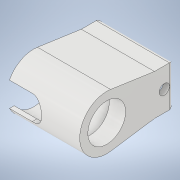
# Autodesk Inventor part: tail_encoder
Saved by Autodesk Inventor 2020 (Build 240168000, 168)
## iProperties
Created: 2018-05-10
Part Number: tail_encoder
Material: Generic
Document SubType Name: Modeling
Designer: stedrock
Density: 1 g/cm^3
Appearance: Default
Mass: 13.8851 g
Surface Area: 94.7181 cm^2
Volume: 13.8851 cm^3
PCB_thickness: 1.650 mm
wall: 3.000 mm
PCB_height: 3.460 mm
Author: stedrock
Autodesk Inventor part; units mm, degrees
sketch "Sketch1" plane through (0, 0, 0) normal (0, 0, 1) x (1, 0, 0)
  line L0 (-9.42, -6.99) -> (9.42, -6.99)
  line L1 (9.42, -6.99) -> (9.42, 6.99)
  line L2 (9.42, 6.99) -> (-9.42, 6.99)
  line L3 (-9.42, 6.99) -> (-9.42, -6.99)
  line L4 (-9.42, -6.99) -> (9.42, 6.99) construction
  line L5 (9.42, -6.99) -> (-9.42, 6.99) construction
  line L6 (0, 0) -> (-12.7572, 0) construction
  line L7 (-4.42, -2.5) -> (1.88, -2.5)
  line L8 (1.88, -2.5) -> (1.88, 2.5)
  line L9 (1.88, 2.5) -> (-4.42, 2.5)
  line L10 (-4.42, 2.5) -> (-4.42, -2.5)
  line L11 (-4.42, -2.5) -> (1.88, 2.5) construction
  line L12 (1.88, -2.5) -> (-4.42, 2.5) construction
  line L13 (-12.42, -9.99) -> (23.42, -9.99)
  line L14 (23.42, -9.99) -> (23.42, 9.99)
  line L15 (23.42, 9.99) -> (-12.42, 9.99)
  line L16 (-12.42, 9.99) -> (-12.42, -9.99)
  line L17 (-12.42, -9.99) -> (23.42, 9.99) construction
  line L18 (23.42, -9.99) -> (-12.42, 9.99) construction
  line L19 (-9.42, 6.99) -> (-7.42, 6.99)
  line L20 (-7.42, 6.99) -> (-7.42, -6.99)
  line L21 (-7.42, -6.99) -> (-9.42, -6.99)
  line L22 (-9.42, -6.99) -> (-9.42, 6.99)
  line L23 (-9.42, 6.99) -> (5.42, 6.99)
  line L24 (5.42, 6.99) -> (5.42, 4.99)
  line L25 (5.42, 4.99) -> (-9.42, 4.99)
  line L26 (-9.42, 4.99) -> (-9.42, 6.99)
  line L27 (-9.42, -6.99) -> (5.42, -6.99)
  line L28 (5.42, -6.99) -> (5.42, -4.99)
  line L29 (5.42, -4.99) -> (-9.42, -4.99)
  line L30 (-9.42, -4.99) -> (-9.42, -6.99)
  line L31 (-1.27, 0) -> (31.11, 0) construction
  line L32 (9.42, 6.99) -> (20.42, 6.99)
  line L33 (20.42, 6.99) -> (20.42, -6.99)
  line L34 (20.42, -6.99) -> (9.42, -6.99)
  line L35 (9.42, -6.99) -> (9.42, 6.99)
  line L36 (9.42, 6.99) -> (20.42, -6.99) construction
  line L37 (20.42, 6.99) -> (9.42, -6.99) construction
  circle A0 centre (-1.27, 0) radius 1.5
  line L38 (19.42, -6.99) -> (19.42, 6.99)
  point P0 (5.5, 0)
  point P1 (14.92, 0)
  dimension "d0" = 18.84
  dimension "d1" = 13.98
  dimension "d2" = 6.3
  dimension "d3" = 5
  dimension "d4" = 11.3
  dimension "d5" = 13.84
  dimension "d10" = 3
  dimension "d11" = 3
  dimension "d12" = 14
  dimension "d17" = 2
  dimension "d18" = 2
  dimension "d19" = 4
  dimension "d20" = 2
  dimension "d21" = 4
  dimension "d22" = 3
  dimension "d25" = 3
  dimension "d47" = 10
  constraints: 78 end point, 14 parallel, 9 midpoint, 8 perpendicular, 7 horizontal, 6 point on line, 1 centre point, 1 coincident, 1 vertical
  measures "d0" distance of L2.end L1.end
  measures "d1" distance of L1.end L0.end
  measures "d2" distance of L9.end L8.end
  measures "d3" distance of L7.end L8.end
  measures "d4" distance between parallel lines of L8 L3
  measures "d5" distance between parallel lines of L1 L10
  measures "d10" distance between parallel lines of L2 L15
  measures "d11" distance between parallel lines of L3 L16
  measures "d12" distance between parallel lines of L14 L1
  measures "d17" distance between parallel lines of L20 L3
  measures "d18" distance of L23.end L24.end
  measures "d19" distance between parallel lines of L1 L24
  measures "d20" distance between parallel lines of L27 L29
  measures "d21" distance between parallel lines of L1 L28
  measures "d22" distance between parallel lines of L14 L33
  measures "d25" diameter of A0
  measures "d47" distance between parallel lines of L38 L35
extrude "top" add sketch "Sketch1" against normal blind 7 contours L16 L15 L14 L13
extrude "bottom" add sketch "Sketch1" along normal blind 2.31 contours L3 L29 L20 L0 | L20 L29 L28 L0 | L3 L25 L20 L29 | L3 L2 L20 L25 | L20 L2 L24 L25 | L38 L32 L33 L34 | L16 L15 L14 L13
ref_plane "Work Plane1" through (23.42, 9.99, 0) normal (1, 0, 0) x (0, 1, 0)
sketch "Sketch2" plane through (23.42, 9.99, 0) normal (1, 0, 0) x (0, 1, 0)
  line L0 (-9.99, 0) -> (-9.99, 39.738) construction
  circle A0 centre (-9.99, 25.712) radius 9.25
  circle A1 centre (-9.99, 25.712) radius 13.25
  line L1 (-19.98, 0) -> (0, 0) projected
  line L2 (-19.98, 2.31) -> (0, 2.31) projected
  line L3 (0, 2.31) -> (3.1224, 23.8075)
  line L4 (-19.98, 2.31) -> (-23.1024, 23.8075)
  line L5 (-6.699, 7.9835) -> (-13.281, 7.9835) construction
  line L6 (-6.699, 10.4835) -> (-13.281, 10.4835)
  line L7 (-13.281, 5.4835) -> (-6.699, 5.4835)
  arc A2 (-6.699, 5.4835) -> (-6.699, 10.4835) centre (-6.699, 7.9835) ccw
  arc A3 (-13.281, 10.4835) -> (-13.281, 5.4835) centre (-13.281, 7.9835) ccw
  circle A4 centre (-9.99, -2.5) radius 2.5
  point P0 (-9.99, 7.9835)
  dimension "d26" = 18.5
  dimension "d27" = 26.5
  dimension "d30" = 23.402
  dimension "d33" = 5
  dimension "d43" = 5
  dimension "d44" = 2.5
  constraints: 14 end point, 6 point on circle, 6 tangent, 5 centre point, 3 point on line, 1 coincident, 1 midpoint, 1 parallel, 1 perpendicular, 1 vertical
  measures "d26" diameter of A0
  measures "d27" diameter of A1
  measures "d30" distance from line of A0.centre L2
  measures "d33" diameter of A3
  measures "d43" diameter of A4
  measures "d44" distance from line of L1 A4.centre
extrude "holder" add sketch "Sketch2" against normal blind 8 contours A1 | A1 L3 L2 L4 | A2 L7 A3 L6
sketch "Sketch4" plane through (15.42, 9.99, 0) normal (-1, 0, 0) x (0, 0, 1)
  circle A0 centre (25.712, -9.99) radius 9.25 projected
  line L0 (23.8075, 3.1224) -> (2.31, 0) projected
  line L1 (2.31, -19.98) -> (23.8075, -23.1024) projected
  circle A1 centre (25.712, -9.99) radius 11.25
  line L2 (2.31, -19.98) -> (2.31, 0) projected
  arc A2 (23.8075, -23.1024) -> (23.8075, 3.1224) centre (25.712, -9.99) ccw projected
  line L3 (2.31, 0) -> (2.31, -19.98) projected
  line L4 (2.31, -16.9485) -> (19.65, -19.4671)
  line L5 (2.31, -3.0315) -> (19.65, -0.5129)
  circle A3 centre (25.712, -9.99) radius 13.25 projected
  line L6 (12.462, -1.5569) -> (12.462, -18.4231)
  point P0 (0, -9.99)
  point P1 (2.31, -2.0103)
  point P2 (24.5722, 1.2021)
  point P3 (2.31, -18.1795)
  point P4 (29.9517, -20.4105)
  dimension "d34" = 22.5
  dimension "d41" = 3
  dimension "d42" = 3
  constraints: 6 end point, 6 point on line, 4 point on circle, 2 parallel, 1 centre point, 1 coincident, 1 tangent, 1 vertical
  measures "d34" diameter of A1
  measures "d41" distance between parallel lines of L4 L1
  measures "d42" distance between parallel lines of L0 L5
extrude "holder2" add sketch "Sketch4" along normal up to surface (27.84 mm away) contours A3 L5 L2 L0 | A2 A3 L4 A1 L5 | A3 L6 L5 | L5 A1 L4 A3 | L1 L2 L4 A3 | A3 L4 L6
ref_plane "Work Plane2" through (0, 0, 42.8625) normal (0, 0, 1) x (1, 0, 0)
sketch "Sketch5" plane through (0, 0, 42.8625) normal (0, 0, 1) x (1, 0, 0)
  line L0 (-25.4872, 0) -> (-1.2329, 0) construction
  line L1 (-25.4872, -6) -> (-1.2329, -6)
  line L2 (-1.2329, 6) -> (-25.4872, 6)
  arc A0 (-25.4872, 6) -> (-25.4872, -6) centre (-25.4872, 0) ccw
  arc A1 (-1.2329, -6) -> (-1.2329, 6) centre (-1.2329, 0) ccw
  point P0 (0, 0)
  point P1 (-13.3601, 0)
  dimension "d38" = 12
  constraints: 8 end point, 4 point on circle, 4 tangent, 2 centre point, 1 horizontal, 1 midpoint, 1 parallel, 1 point on line
  measures "d38" diameter of A1
extrude "bottom hole" cut sketch "Sketch5" against normal blind 33.35
extrude "cable hole" cut sketch "Sketch2" against normal up to next contours A4
fillet "Fillet1" radius 2 4 edges at (5.5, 9.99, -7) (23.42, 0, -7) (5.5, -9.99, -7) (-12.42, 0, -7)
ref_plane "trim plane" through (-12.42, 9.99, 2.31) normal (0, 0, 1) x (1, 0, 0)
ref_plane "Work Plane4" through (47.625, 0, 0) normal (1, 0, 0) x (0, 1, 0)
sketch "split sketch" plane through (47.625, 0, 0) normal (1, 0, 0) x (0, 1, 0)
  line L0 (9.99, -5) -> (0, -5) projected
  line L1 (9.99, -5) -> (9.99, 2.31) projected
  line L2 (9.99, 2.31) -> (13.1124, 23.8075) projected
  arc A0 (13.1124, 23.8075) -> (-13.1124, 23.8075) centre (0, 25.712) ccw projected
  line L3 (-13.1124, 23.8075) -> (-9.99, 2.31) projected
  line L4 (-9.99, -5) -> (-9.99, 2.31) projected
  circle A1 centre (0, -2.5) radius 2.5 projected
  circle A2 centre (0, 25.712) radius 9.25 projected
  line L5 (9.99, -5) -> (9.99, 2.31) projected
  line L6 (-9.99, 2.31) -> (-7.7245, 2.31) projected
  line L7 (9.99, 2.31) -> (-9.99, 2.31)
  line L8 (9.99, 2.31) -> (-9.99, 2.31) projected
  line L9 (7.99, 2.31) -> (-7.99, 2.31)
  line L10 (-7.99, 2.31) -> (-7.99, -12.786)
  line L11 (-7.99, -12.786) -> (7.99, -12.786)
  line L12 (7.99, -12.786) -> (7.99, 2.31)
  line L13 (26.885, -21.7939) -> (-23.4802, -21.7939)
  line L14 (-23.4802, -21.7939) -> (-23.4802, 46.6825)
  line L15 (-23.4802, 46.6825) -> (26.885, 46.6825)
  line L16 (26.885, 46.6825) -> (26.885, -21.7939)
  line L17 (-9.99, -5) -> (9.99, -5) projected
  line L18 (0, -5) -> (-9.99, -5) projected
  line L19 (-7.99, -5) -> (-9.99, -5)
  line L20 (-9.99, -5) -> (-9.99, 2.31)
  line L21 (-9.99, 2.31) -> (-7.99, 2.31)
  line L22 (-7.99, 2.31) -> (-7.99, -5)
  line L23 (9.99, -5) -> (9.99, 2.31) projected
  line L24 (7.99, -5) -> (9.99, -5)
  line L25 (9.99, -5) -> (9.99, 2.31)
  line L26 (9.99, 2.31) -> (7.99, 2.31)
  line L27 (7.99, 2.31) -> (7.99, -5)
  point P0 (0, 0)
  dimension "d52" = 2
  dimension "d53" = 2
  constraints: 34 end point, 8 parallel, 5 horizontal, 5 point on line, 4 perpendicular, 1 vertical alignment
  measures "d52" distance between parallel lines of L12 L1
  measures "d53" distance between parallel lines of L4 L10
extrude "top part" [suppressed]
extrude "bottom part" [suppressed]
equation "\"d10\" = wall"
equation "\"d11\" = wall"
equation "\"d20\" = d18"
equation "\"d21\" = d19"
equation "\"d22\" = wall"
equation "\"d44\" = 0.5 * d43"
equation "\"d42\" = d41"
equation "\"d53\" = d52"
equation "\"PCB_thickness\" = 1.65"
equation "\"wall\" = 3"
equation "\"PCB_height\" = 3.46"
body "Solid2"
